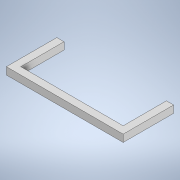
# Autodesk Inventor part: BatteryHolder
Saved by Autodesk Inventor 2022 (Build 260153000, 153)
## iProperties
Created: 2022-01-11
Part Number: BatteryHolder
Material: Generic
Document SubType Name: Modeling
Designer: Daniel Marquez
Density: 1 g/cm^3
Appearance: Default
Author: Daniel Marquez
Autodesk Inventor part; units mm, degrees
ref_plane "YZ Plane" through (0, 0, 0) normal (1, 0, 0) x (0, 1, 0)
ref_plane "XZ Plane" through (0, 0, 0) normal (0, 1, 0) x (-1, 0, 0)
ref_plane "XY Plane" through (0, 0, 0) normal (0, 0, 1) x (1, 0, 0)
sketch "Sketch2" plane through (0, 0, 0) normal (0, 1, 0) x (-1, 0, 0)
  line L0 (-180.34, -76.2) -> (-180.34, 0)
  line L1 (-193.04, 0) -> (-193.04, -76.2)
  line L2 (-193.04, -76.2) -> (-180.34, -76.2)
  line L3 (-180.34, -76.2) -> (-180.34, 0)
  line L4 (0, -76.2) -> (-180.34, -76.2)
  line L5 (0, -76.2) -> (12.7, -76.2)
  line L6 (12.7, -76.2) -> (12.7, 0)
  line L7 (0, 0) -> (0, -76.2)
  line L8 (0, 0) -> (-180.34, 0)
  line L9 (-193.04, 0) -> (-193.04, 12.7)
  line L10 (-193.04, 12.7) -> (12.7, 12.7)
  line L11 (12.7, 12.7) -> (12.7, 0)
  dimension "d8" = 12.7
  dimension "d9" = 12.7
  dimension "d10" = 12.7
  constraints: 24 end point, 4 parallel, 2 horizontal, 2 perpendicular, 1 point on line
  measures "d8" distance of L2.end L1.end
  measures "d9" distance of L7.start L6.end
  measures "d10" distance of L9.start L9.end
extrude "Extrusion2" add sketch "Sketch2" along normal blind 12.7 contours L2 L1 L9 L10 L11 L6 L5 L7 L8 L0
body "Solid2"
